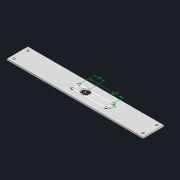
# Autodesk Inventor part: s_carbon_plate3
Saved by Autodesk Inventor 2021 (Build 250183000, 183)
## iProperties
Created: 2021-08-20
Part Number: s_carbon_plate3
Material: 一般
Document SubType Name: Sheet Metal
Designer: yuta0
Density: 1 g/cm^3
Sheet Metal Rule: Default_mm
Appearance: 既定
Author: yuta0
Autodesk Inventor part; units mm, degrees
ref_plane "YZ Plane" through (0, 0, 0) normal (1, 0, 0) x (0, 1, 0)
ref_plane "XZ Plane" through (0, 0, 0) normal (0, 1, 0) x (-1, 0, 0)
ref_plane "XY Plane" through (0, 0, 0) normal (0, 0, 1) x (1, 0, 0)
sketch "スケッチ1" plane through (0, 0, 0) normal (0, 1, 0) x (-1, 0, 0)
  line L0 (97.5, 15) -> (-97.5, 15)
  line L1 (-97.5, 15) -> (-97.5, -15)
  line L2 (-97.5, -15) -> (97.5, -15)
  line L3 (97.5, -15) -> (97.5, 15)
  line L4 (97.5, 15) -> (-97.5, -15) construction
  line L5 (-97.5, 15) -> (97.5, -15) construction
  point P0 (0, 0)
  dimension "d0" = 195
  dimension "d1" = 30
  measures "d0" distance of L1.end L2.end
  measures "d1" distance of L2.end L0.start
extrude "プレート1" add sketch "スケッチ1" along normal blind 2
sketch "スケッチ2" plane through (0, 2, 0) normal (0, 1, 0) x (1, 0, 0)
  line L0 (-14, -5) -> (34.6, -5)
  line L1 (34.6, -5) -> (34.6, 5)
  line L2 (34.6, 5) -> (-14, 5)
  line L3 (-14, 5) -> (-14, -5)
  line L4 (-14, -5) -> (34.6, 5) construction
  line L5 (34.6, -5) -> (-14, 5) construction
  point P0 (0, 0)
  point P1 (10.3, 0)
  point P2 (10.3, 0)
  dimension "d3" = 48.6
  dimension "d4" = 14
  dimension "d5" = 10
  constraints: 12 end point, 3 midpoint, 2 parallel, 1 horizontal, 1 horizontal alignment, 1 perpendicular
  measures "d3" distance of L1.end L2.end
  measures "d4" distance from line of L3 point (0, 0)
  measures "d5" distance of L0.end L1.end
hole "穴1" at (34.6, 2, -5) at (34.6, 2, 5) at (-14, 2, -5) at (-14, 2, 5) direction (0, -1, 0) diameter 4.3 end through all clearance for "Socket Head Cap Screw" size "M4" standard "Ansi Metric M Profile"
sketch "スケッチ3" plane through (0, 2, 0) normal (0, 1, 0) x (1, 0, 0)
  circle A0 centre (0, 0) radius 6
  dimension "d13" = 12
  constraints: 1 centre point, 1 coincident
  measures "d13" diameter of A0
extrude "押し出し1" cut sketch "スケッチ3" against normal through all
sketch "スケッチ4" plane through (0, 2, 0) normal (0, 1, 0) x (1, 0, 0)
  line L0 (97.5, 15) -> (97.5, -15) projected
  line L1 (-97.5, 15) -> (97.5, 15) projected
  line L2 (97.5, -15) -> (-97.5, -15) projected
  line L3 (-97.5, -15) -> (-97.5, 15) projected
  point P0 (0, 0)
  point P1 (-92.5, 10)
  point P2 (-92.5, -10)
  point P3 (92.5, 10)
  point P4 (92.5, -10)
  dimension "d16" = 5
  dimension "d17" = 5
  dimension "d18" = 5
  dimension "d19" = 5
  constraints: 2 horizontal alignment, 2 vertical alignment
  measures "d16" distance from line of L0 point (92.5, 10)
  measures "d17" distance from line of L1 point (92.5, 10)
  measures "d18" distance from line of L2 point (92.5, -10)
  measures "d19" distance from line of L3 point (-92.5, 10)
hole "穴2" at (-92.5, 2, -10) at (-92.5, 2, 10) at (92.5, 2, -10) at (92.5, 2, 10) direction (0, -1, 0) diameter 3.2 end through all clearance for "Socket Head Cap Screw" size "M3" standard "Ansi Metric M Profile"
equation "\"d11\" = Thickness"
equation "\"d25\" = Thickness"
equation "\"d2\" = Thickness"
equation "\"BendRadius\" = Thickness"
equation "\"BendReliefWidth\" = Thickness"
equation "\"BendReliefDepth\" = 0.5 * Thickness"
equation "\"CornerReliefSize\" = 4 * Thickness"
equation "\"MinimumRemnant\" = 2 * Thickness"
equation "\"TransitionRadius\" = BendRadius"
equation "\"JacobiRadiusSize\" = BendRadius"
equation "\"GapSize\" = Thickness"
equation "\"Thickness\" = 2"
